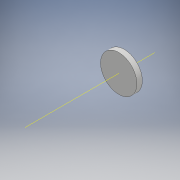
# Autodesk Inventor part: 镜头
Saved by Autodesk Inventor 2017 (Build 210142000, 142)
## iProperties
Part Number: 镜头
Material: 常规
Document SubType Name: Modeling
Designer: Administrator
Density: 1 g/cm^3
Appearance: 默认
Author: Administrator
Autodesk Inventor part; units mm, degrees
ref_plane "YZ Plane" through (0, 0, 0) normal (1, 0, 0) x (0, 1, 0)
ref_plane "XZ Plane" through (0, 0, 0) normal (0, 1, 0) x (-1, 0, 0)
ref_plane "XY Plane" through (0, 0, 0) normal (0, 0, 1) x (1, 0, 0)
sketch "草图1" plane through (0, 0, 0) normal (0, 1, 0) x (-1, 0, 0)
  circle A0 centre (0, 0) radius 6
  dimension "d0" = 12
  constraints: 1 centre point, 1 coincident
  measures "d0" diameter of A0
extrude "拉伸1" add sketch "草图1" along normal blind 1.8
sketch "草图2" plane through (0, 0, 0) normal (1, 0, 0) x (0, 1, 0)
  line L0 (1.8, -6) -> (1.8, 6) projected
  line L1 (1.8, 0) -> (2.3, 0)
  line L2 (1.8, 0) -> (1.8, -6)
  line L3 (0, -6) -> (1.8, -6) projected
  arc A0 (1.8, -6) -> (2.3, 0) centre (-27.6955, -0.5212) ccw
  line L4 (-33.5251, 0) -> (8.6824, 0) projected
  point P0 (0, 0)
  dimension "d3" = 0.5
  dimension "d4" = 30
  constraints: 4 end point, 2 point on circle, 1 centre point, 1 horizontal, 1 midpoint, 1 perpendicular
  measures "d3" distance of L1.start L1.end
  measures "d4" radius of A0
revolve "旋转1" add sketch "草图2" angle 360 about axis through (0, 0, 0) along (0, 1, 0)
